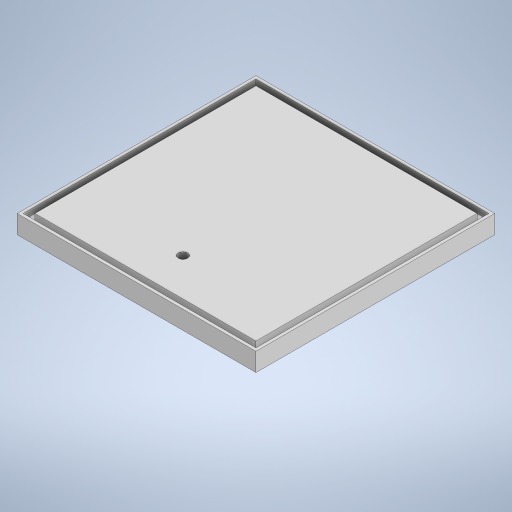
# Autodesk Inventor part: 사각형 OV-PAM 5패턴 상단
Saved by Autodesk Inventor 2024 (Build 280153000, 153)
## iProperties
Created: 2023-06-16
Part Number: 사각형 OV-PAM 5패턴 상단
Material: 일반
Document SubType Name: Modeling
Designer: jsw
Density: 1 g/cm^3
Appearance: 기본값
Author: jsw
Autodesk Inventor part; units mm, degrees
ref_plane "YZ Plane" through (0, 0, 0) normal (1, 0, 0) x (0, 1, 0)
ref_plane "XZ Plane" through (0, 0, 0) normal (0, 1, 0) x (-1, 0, 0)
ref_plane "XY Plane" through (0, 0, 0) normal (0, 0, 1) x (1, 0, 0)
sketch "스케치1" plane through (0, 0, 0) normal (0, 1, 0) x (-1, 0, 0)
  line L0 (-30, 30) -> (30, 30)
  line L1 (30, 30) -> (30, -30)
  line L2 (30, -30) -> (-30, -30)
  line L3 (-30, -30) -> (-30, 30)
  line L4 (-30, 30) -> (30, -30) construction
  line L5 (30, 30) -> (-30, -30) construction
  line L6 (-32.4, 32.4) -> (32.4, 32.4)
  line L7 (32.4, 32.4) -> (32.4, -32.4)
  line L8 (32.4, -32.4) -> (-32.4, -32.4)
  line L9 (-32.4, -32.4) -> (-32.4, 32.4)
  line L10 (-32.4, 32.4) -> (32.4, -32.4) construction
  line L11 (32.4, 32.4) -> (-32.4, -32.4) construction
  point P0 (0, 0)
  dimension "d45" = 60
  dimension "d46" = 60
  dimension "d47" = 2.4
  constraints: 24 end point, 4 midpoint, 4 parallel, 2 horizontal, 2 perpendicular, 1 point on line
  measures "d45" distance of L1.end L2.end
  measures "d46" distance of L2.end L0.start
  measures "d47" distance between parallel lines of L2 L8
extrude "돌출7" add sketch "스케치1" along normal blind 5 contours L0 L1 L2 L3 | L6 L7 L8 L9
sketch "스케치7" plane through (0, 5, 0) normal (0, 1, 0) x (1, 0, 0)
  line L0 (-30, -30) -> (30, -30)
  line L1 (30, -30) -> (30, 30)
  line L2 (30, 30) -> (-30, 30)
  line L3 (-30, 30) -> (-30, -30)
  line L4 (-30, -30) -> (30, 30) construction
  line L5 (30, -30) -> (-30, 30) construction
  line L6 (31.6, -31.6) -> (-31.6, -31.6)
  line L7 (-31.6, -31.6) -> (-31.6, 31.6)
  line L8 (-31.6, 31.6) -> (31.6, 31.6)
  line L9 (31.6, 31.6) -> (31.6, -31.6)
  line L10 (31.6, -31.6) -> (-31.6, 31.6) construction
  line L11 (-31.6, -31.6) -> (31.6, 31.6) construction
  point P0 (0, 0)
  dimension "d50" = 60
  dimension "d51" = 60
  dimension "d52" = 1.6
  constraints: 24 end point, 4 midpoint, 4 parallel, 2 horizontal, 2 perpendicular, 1 point on line
  measures "d50" distance of L1.end L2.end
  measures "d51" distance of L0.end L1.end
  measures "d52" distance between parallel lines of L2 L8
extrude "돌출8" cut sketch "스케치7" against normal blind 1.6
sketch "스케치8" plane through (0, 0, 0) normal (0, -1, 0) x (1, 0, 0)
  line L0 (-20, -2.5) -> (-10, -2.5)
  line L1 (-10, -2.5) -> (-10, 2.5)
  line L2 (-10, 2.5) -> (-20, 2.5)
  line L3 (-20, 2.5) -> (-20, -2.5)
  line L4 (-20, -2.5) -> (-10, 2.5) construction
  line L5 (-10, -2.5) -> (-20, 2.5) construction
  line L6 (10, -2.5) -> (20, -2.5)
  line L7 (20, -2.5) -> (20, 2.5)
  line L8 (20, 2.5) -> (10, 2.5)
  line L9 (10, 2.5) -> (10, -2.5)
  line L10 (10, -2.5) -> (20, 2.5) construction
  line L11 (20, -2.5) -> (10, 2.5) construction
  line L12 (32.4, 32.4) -> (32.4, -32.4) projected
  line L13 (32.4, 0) -> (20, 0)
  line L14 (-20, 0) -> (-32.4, 0)
  line L15 (-32.4, -32.4) -> (-32.4, 32.4) projected
  point P0 (0, 0)
  point P1 (-15, 0)
  point P2 (15, 0)
  dimension "d55" = 10
  dimension "d56" = 5
  dimension "d57" = 20
  dimension "d58" = 10
  dimension "d61" = 12.4
  constraints: 28 end point, 8 midpoint, 4 parallel, 2 horizontal, 2 horizontal alignment, 2 perpendicular, 1 point on line
  measures "d55" distance of L1.end L2.end
  measures "d56" distance of L2.end L0.start
  measures "d57" distance between parallel lines of L9 L1
  measures "d58" distance of L6.start L6.end
  measures "d61" distance between parallel lines of L7 L12
extrude "돌출9" add sketch "스케치8" along normal blind 10
sketch "스케치9" plane through (-10, 0, -2.5) normal (0, 0, -1) x (-1, 0, 0)
  line L0 (10, -10) -> (0, -10) projected
  circle A0 centre (5, -10) radius 5
  line L1 (-20, -10) -> (-30, -10) projected
  circle A1 centre (-25, -10) radius 5
  point P0 (-10, 0)
  dimension "d64" = 10
  dimension "d65" = 10
  constraints: 2 centre point, 2 midpoint
  measures "d64" diameter of A0
  measures "d65" diameter of A1
extrude "돌출10" add sketch "스케치9" against normal blind 5
sketch "스케치10" plane through (-10, 0, -2.5) normal (0, 0, -1) x (-1, 0, 0)
  arc A0 (0, -10) -> (10, -10) centre (5, -10) ccw projected
  circle A1 centre (5, -10) radius 1.25
  arc A2 (-30, -10) -> (-20, -10) centre (-25, -10) ccw projected
  circle A3 centre (-25, -10) radius 1.25
  point P0 (-10, 0)
  dimension "d68" = 2.5
  dimension "d69" = 2.5
  constraints: 2 centre point, 2 coincident
  measures "d68" diameter of A1
  measures "d69" diameter of A3
extrude "돌출11" cut sketch "스케치10" against normal blind 5
sketch "스케치11" plane through (0, 0, 0) normal (0, -1, 0) x (1, 0, 0)
  circle A0 centre (0, 19.821) radius 1.25
  line L0 (-20, 2.5) -> (-10, 2.5) projected
  point P0 (0, 0)
  dimension "d72" = 2.5
  dimension "d73" = 17.321
  constraints: 1 centre point, 1 vertical alignment
  measures "d72" diameter of A0
  measures "d73" distance from line of A0.centre L0
extrude "돌출12" cut sketch "스케치11" against normal blind 5
